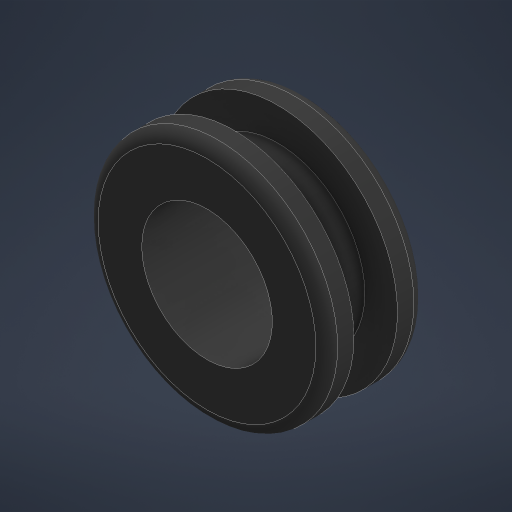
# Autodesk Inventor part: Tarot_12mm_Rubber
Saved by Autodesk Inventor 2024 (Build 280153000, 153)
## iProperties
Created: 2023-06-28
Part Number: Tarot_12mm_Rubber
Material: Rubber
Document SubType Name: Modeling
Designer: dzw04
Density: 0.93 g/cm^3
Appearance: Rubber - Black
Author: dzw04
Autodesk Inventor part; units mm, degrees
ref_plane "YZ Plane" through (0, 0, 0) normal (1, 0, 0) x (0, 1, 0)
ref_plane "XZ Plane" through (0, 0, 0) normal (0, 1, 0) x (-1, 0, 0)
ref_plane "XY Plane" through (0, 0, 0) normal (0, 0, 1) x (1, 0, 0)
sketch "Sketch1" plane through (0, 0, 0) normal (0, 1, 0) x (-1, 0, 0)
  line L0 (0, 0) -> (6, 0) construction
  line L1 (6, 0) -> (11, 0) construction
  line L2 (6, 0) -> (6, -4.5)
  line L3 (6, -4.5) -> (10, -4.5)
  line L4 (11, -3.5) -> (11, -2)
  line L5 (11, -2) -> (8, -2)
  line L6 (8, -2) -> (8, 0)
  arc A0 (10, -4.5) -> (11, -3.5) centre (10, -3.5) ccw
  line L7 (6, 0) -> (6, 4.5)
  line L8 (6, 4.5) -> (10, 4.5)
  line L9 (11, 3.5) -> (11, 2)
  line L10 (11, 2) -> (8, 2)
  line L11 (8, 2) -> (8, 0)
  arc A1 (11, 3.5) -> (10, 4.5) centre (10, 3.5) ccw
  line L12 (0, -6.5899) -> (0, 6.5899) projected
  point P0 (11, -4.5)
  point P1 (11, 4.5)
  dimension "d0" = 6
  dimension "d1" = 5
  dimension "d2" = 4.5
  dimension "d3" = 5
  dimension "d4" = 2.5
  dimension "d5" = 3
  dimension "d6" = 1
  constraints: 24 end point, 7 symmetric about line, 6 point on line, 4 point on circle, 3 perpendicular, 2 centre point, 2 horizontal, 2 tangent, 1 vertical, 1 other
  measures "d0" distance of L0.start L0.end
  measures "d1" distance of L0.end L1.end
  measures "d2" distance of L0.end L2.end
  measures "d3" distance of L2.end point (11, -4.5)
  measures "d4" distance of point (11, -4.5) L4.end
  measures "d5" distance of L4.end L5.end
  measures "d6" radius of A0
revolve "Revolution1" add sketch "Sketch1" angle 360 about axis through (0, 0, -10) along (0, 0, 1)
body "Solid1"
